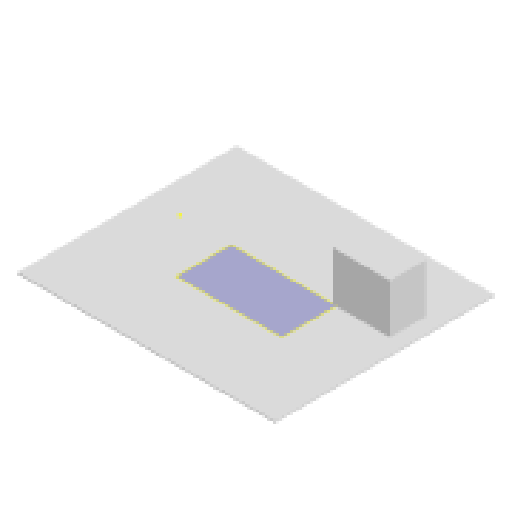
# Autodesk Inventor part: Земля_и_Препятствия
Saved by Autodesk Inventor 2026 (Build 300175000, 175)
## iProperties
Created: 2026-05-26
Part Number: Земля_и_Препятствия
Material: Типовые
Document SubType Name: Modeling
Designer: Artem Sannikov
Density: 1 g/cm^3
Appearance: По умолчанию
Author: Artem Sannikov
Autodesk Inventor part; units mm, degrees
ref_plane "YZ Plane" through (0, 0, 0) normal (1, 0, 0) x (0, 1, 0)
ref_plane "XZ Plane" through (0, 0, 0) normal (0, 1, 0) x (-1, 0, 0)
ref_plane "XY Plane" through (0, 0, 0) normal (0, 0, 1) x (1, 0, 0)
ref_plane "РабПлоскость1" through (475.3287, -140.8035, 12.4703) normal (0, -1, 0) x (1, 0, 0)
sketch "Эскиз1" plane through (475.3287, -140.8035, 12.4703) normal (0, -1, 0) x (1, 0, 0)
  point P0 (-475.3287, -12.4703)
sketch "Эскиз2" plane through (475.3287, -140.8035, 12.4703) normal (0, -1, 0) x (1, 0, 0)
  line L0 (-735.7265, 1024.2535) -> (1318.2521, 1024.2535)
  line L1 (1318.2521, 1024.2535) -> (1318.2521, -723.0885)
  line L2 (1318.2521, -723.0885) -> (-735.7265, -723.0885)
  line L3 (-735.7265, -723.0885) -> (-735.7265, 1024.2535)
  point P0 (-475.3287, -12.4703)
  constraints: 8 end point, 2 parallel, 1 horizontal, 1 perpendicular
extrude "Выдавливание1" add sketch "Эскиз2" along normal blind 10
sketch "Эскиз3" plane through (475.3287, -140.8035, 12.4703) normal (0, 1, 0) x (1, 0, 0)
  line L0 (1194.1306, 12.4703) -> (738.2489, 12.4703)
  line L1 (738.2489, 12.4703) -> (738.2489, 295.0097)
  line L2 (738.2489, 295.0097) -> (1194.1306, 295.0097)
  line L3 (1194.1306, 295.0097) -> (1194.1306, 12.4703)
  point P0 (-475.3287, 12.4703)
  constraints: 8 end point, 2 parallel, 1 horizontal, 1 perpendicular
extrude "Выдавливание2" add sketch "Эскиз3" along normal blind 390
sketch "Эскиз4" plane through (475.3287, -140.8035, 12.4703) normal (0, 1, 0) x (1, 0, 0)
  line L0 (1194.1306, 295.0097) -> (1194.1306, 12.4703) projected
  line L1 (1194.1306, 12.4703) -> (738.2489, 12.4703) projected
  line L2 (738.2489, 12.4703) -> (738.2489, 295.0097) projected
  line L3 (738.2489, 295.0097) -> (1194.1306, 295.0097) projected
  line L4 (-735.7265, 723.0885) -> (1318.2521, 723.0885) projected
  line L5 (-735.7265, -1024.2535) -> (-735.7265, 723.0885) projected
  line L6 (1318.2521, -1024.2535) -> (-735.7265, -1024.2535) projected
  line L7 (1318.2521, 723.0885) -> (1318.2521, -1024.2535) projected
  point P0 (-475.3287, 12.4703)
extrude "Выдавливание3" add sketch "Эскиз4" along normal blind 50.25
